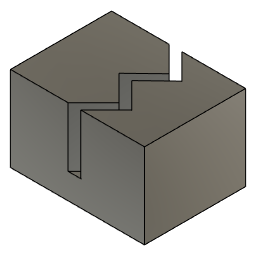
Držák řemene v3 (Autodesk Fusion 360 design; units mm, degrees)
Autodesk Fusion 360 part; units mm, degrees
sketch "Sketch6" plane through (0, 0, 0) normal (0, 0, 1) x (1, 0, 0)
  line L0 (78, 1.6) -> (70.5, 1.6)
  line L1 (69, 13.5) -> (72, 10.5)
  line L2 (72, 10.5) -> (69, 7.6)
  line L3 (69, 7.6) -> (72, 4.6)
  line L4 (72, 4.6) -> (69, 1.6)
  line L5 (70.5, 13.5) -> (73.5, 10.5)
  line L6 (73.5, 10.5) -> (70.5, 7.6)
  line L7 (73.5, 4.6) -> (70.5, 1.6)
  line L8 (70.5, 7.6) -> (73.5, 4.6)
  line L9 (69, 13.5) -> (62.2186, 13.5)
  line L10 (62.2186, 13.5) -> (62.2186, 1.6)
  line L11 (69, 1.6) -> (62.2186, 1.6)
  line L12 (70.5, 13.5) -> (78, 13.5)
  line L13 (78, 13.5) -> (78, 1.6)
  line L14 (62.2186, 13.5) -> (78, 13.5)
  line L15 (78, 13.5) -> (78, 1.6)
  line L16 (78, 1.6) -> (62.2186, 1.6)
  line L17 (62.2186, 1.6) -> (62.2186, 13.5)
  constraint horizontal L0
  constraint horizontal L9
  constraint vertical L10
  constraint horizontal L11
  constraint vertical L13
  constraint horizontal L12
  constraint coincident L2.start L1
  constraint coincident L2 L1.end
  constraint coincident L3.start L2
  constraint coincident L3 L2.end
  constraint coincident L4.start L3
  constraint coincident L3.end L4
  constraint coincident L5 L6.start
  constraint coincident L5.end L6
  constraint coincident L6 L8.start
  constraint coincident L6.end L8
  constraint coincident L7.start L8
  constraint coincident L8.end L7
  constraint coincident L11 L10.end
  constraint coincident L10 L11.end
  constraint coincident L10 L9.end
  constraint coincident L10.start L9
  constraint coincident L13 L0.start
  constraint coincident L0 L13.end
  constraint horizontal L14
  constraint vertical L15
  constraint horizontal L16
  constraint vertical L17
extrude "Extrude17" add sketch "Sketch6" along normal blind 3 makes body 1
extrude "Extrude18" add sketch "Sketch6" along normal blind 10 separate body contours L0 L5 L6 L7 L8 L12 L13 L14 L15 L16 | L1 L2 L3 L4 L9 L10 L11 L14 L16 L17 makes body 2 at (78, 9.5333, 3.3333) makes body 3 at (62.2186, 5.5667, 6.6667)
combine "Combine1" operation add target body 1 tool bodies 2 3
extrude "Extrude12" [suppressed]
copy_body "Body->Comp1" [suppressed] in component "Úchytka"
named bodies: "Úchytka", "Základna"
